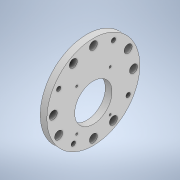
# Autodesk Inventor part: sample-transfer_adapter-plate
Saved by Autodesk Inventor 2020 (Build 240168000, 168)
## iProperties
Created: 2019-08-16
Part Number: sample-transfer_adapter-plate
Material: Generic
Document SubType Name: Modeling
Designer: rainer
Density: 1 g/cm^3
Appearance: Default
Author: rainer
Autodesk Inventor part; units mm, degrees
ref_plane "YZ Plane" through (0, 0, 0) normal (1, 0, 0) x (0, 1, 0)
ref_plane "XZ Plane" through (0, 0, 0) normal (0, 1, 0) x (-1, 0, 0)
ref_plane "XY Plane" through (0, 0, 0) normal (0, 0, 1) x (1, 0, 0)
sketch "Sketch1" plane through (0, 0, 0) normal (1, 0, 0) x (0, 1, 0)
  circle A0 centre (0, 0) radius 34.75
  circle A1 centre (-6.9, 0) radius 14
  dimension "d0" = 69.5
  dimension "d1" = 28
  dimension "d2" = 6.9
  constraints: 2 centre point, 1 coincident
  measures "d0" diameter of A0
  measures "d1" diameter of A1
  measures "d2" distance of point (0, 0) A1.centre
extrude "Extrusion1" add sketch "Sketch1" along normal blind 2
sketch "Sketch2" plane through (0, 0, 0) normal (-1, 0, 0) x (0, 0, 1)
  circle A0 centre (0, 0) radius 30
  line L0 (0, 0) -> (25.9808, 15)
  line L1 (0, 0) -> (30, 0) construction
  dimension "d5" = 60
  dimension "d6" = 30
  constraints: 4 end point, 2 coincident, 1 equal length, 1 horizontal, 3 other
  measures "d6" angle of L1 L0
hole "Hole1" at (0, 15, 25.9808) direction (1, 0, 0) diameter 3.3 depth 5
pattern_circular "Circular Pattern1" count 4 over 360 about axis through (0, 0, 0) along (1, 0, 0) of "Hole1"
thread "Thread1" size "M4x0.7" class "6H" standard "ANSI Metric M Profile" full length
thread "Thread2" size "M4x0.7" class "6H" standard "ANSI Metric M Profile" full length
thread "Thread3" size "M4x0.7" class "6H" standard "ANSI Metric M Profile" full length
thread "Thread4" size "M4x0.7" class "6H" standard "ANSI Metric M Profile" full length
sketch "Sketch3" plane through (2, 0, 0) normal (1, 0, 0) x (0, 0, -1)
  circle A0 centre (0, 0) radius 30
  point P0 (0, 30)
  dimension "d25" = 60
  constraints: 1 coincident, 1 vertical alignment, 2 other
hole "Hole2" at (2, 30, 0) direction (-1, 0, 0) diameter 6 depth 5
pattern_circular "Circular Pattern2" count 4 over 360 about axis through (0, 0, 0) along (1, 0, 0) of "Hole2"
sketch "Sketch4" plane through (0, 0, 0) normal (-1, 0, 0) x (0, 0, 1)
  circle A0 centre (0, 0) radius 30
  line L0 (0, 0) -> (15, 25.9808)
  line L1 (0, 0) -> (30, 0) construction
  point P0 (15, 25.9808)
  dimension "d36" = 60
  dimension "d37" = 60
  constraints: 4 end point, 2 point on circle, 1 centre point, 1 coincident, 1 equal length, 1 horizontal
  measures "d36" diameter of A0
  measures "d37" angle of L1 L0
hole "Hole3" at (0, 25.9808, 15) direction (1, 0, 0) diameter 6 depth 5
pattern_circular "Circular Pattern3" count 4 over 360 about axis through (0, 0, 0) along (1, 0, 0) of "Hole3"
thicken "Thicken1" operation add thickness 3 both sides no extend neighbours yes toward (-1, 0, 0) faces at (0, 19.5446, -6.1067)
sketch "Sketch5" plane through (-3, 0, 0) normal (-1, 0, 0) x (0, 0, 1)
  line L0 (-12.5, 10) -> (12.5, 10)
  line L1 (12.5, 10) -> (12.5, -21)
  line L2 (12.5, -21) -> (-12.5, -21)
  line L3 (-12.5, -21) -> (-12.5, 10)
  point P0 (0, 0)
  point P1 (0, 10)
  dimension "d50" = 25
  dimension "d51" = 10
  dimension "d52" = 31
  constraints: 8 end point, 4 coincident, 2 parallel, 1 horizontal, 1 midpoint, 1 perpendicular, 1 vertical alignment
  measures "d50" distance of L0.start L0.end
  measures "d51" distance from line of point (0, 0) L0
  measures "d52" distance of L0.end L1.end
hole "Hole4" at (-3, 10, -12.5) at (-3, 10, 12.5) at (-3, -21, 12.5) at (-3, -21, -12.5) direction (1, 0, 0) diameter 1.6 depth 5
thread "Thread5" size "M2x0.4" class "6H" standard "ANSI Metric M Profile" full length
thread "Thread6" size "M2x0.4" class "6H" standard "ANSI Metric M Profile" full length
thread "Thread7" size "M2x0.4" class "6H" standard "ANSI Metric M Profile" full length
thread "Thread8" size "M2x0.4" class "6H" standard "ANSI Metric M Profile" full length
body "Solid1"
